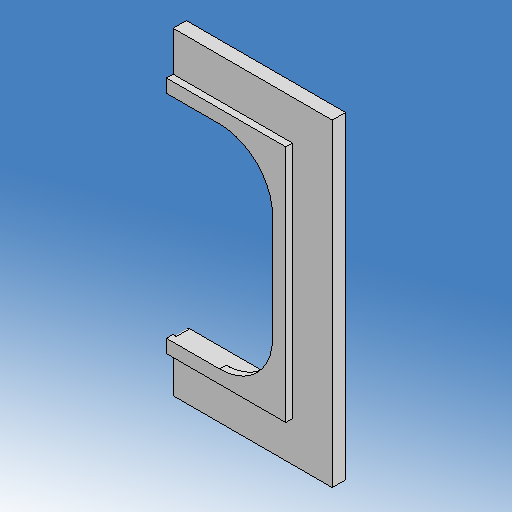
# Autodesk Inventor part: ChassisInterfaceFix
Saved by Autodesk Inventor 2025 (Build 290162000, 162)
## iProperties
Created: 2024-07-07
Part Number: ChassisInterfaceFix
Material: Generic
Document SubType Name: Modeling
Designer: seene
Density: 1 g/cm^3
Appearance: Default
Author: seene
Autodesk Inventor part; units mm, degrees
ref_plane "YZ Plane" through (0, 0, 0) normal (1, 0, 0) x (0, 1, 0)
ref_plane "XZ Plane" through (0, 0, 0) normal (0, 1, 0) x (-1, 0, 0)
ref_plane "XY Plane" through (0, 0, 0) normal (0, 0, 1) x (1, 0, 0)
sketch "Sketch1" plane through (0, 0, 0) normal (0, 0, 1) x (1, 0, 0)
  line L0 (0, 0) -> (76.2, 0)
  line L1 (76.2, 0) -> (76.2, 152.4)
  line L2 (76.2, 152.4) -> (0, 152.4)
  line L3 (0, 152.4) -> (0, 0)
  line L4 (0, 127) -> (50.8, 127)
  line L5 (50.8, 127) -> (50.8, 25.4)
  line L6 (50.8, 25.4) -> (0, 25.4)
  line L7 (0, 25.4) -> (0, 127)
  point P0 (0, 25.4)
  point P1 (76.2, 76.2)
  dimension "d0" = 101.6
  dimension "d1" = 50.8
  dimension "d2" = 25.4
  dimension "d4" = 25.4
  dimension "d9" = 25.4
  constraints: 16 end point, 4 parallel, 2 horizontal, 2 perpendicular, 1 midpoint, 1 point on line
  measures "d0" distance of L4.end L5.end
  measures "d1" distance of L4.start L4.end
  measures "d2" distance between parallel lines of L0 L6
  measures "d4" distance between parallel lines of L4 L2
  measures "d9" distance from line of point (76.2, 76.2) L5
extrude "Extrusion1" add sketch "Sketch1" along normal blind 6.35 contours L3 L6 L5 L4 L2 L1 L0
fillet "Fillet1" radius 12.7 2 edges at (50.8, 127, 3.175) (50.8, 25.4, 3.175)
fillet "Fillet2" radius 1.5875 2 edges at (0, 127, 3.175) (0, 25.4, 3.175)
sketch "Sketch2" plane through (0, 0, 6.35) normal (0, 0, 1) x (1, 0, 0)
  line L0 (0, 127) -> (25.4, 127)
  line L1 (50.8, 101.6) -> (50.8, 50.8)
  line L2 (25.4, 25.4) -> (19.0762, 25.4)
  line L3 (1.5875, 127) -> (38.1, 127) projected
  arc A0 (50.8, 101.6) -> (25.4, 127) centre (25.4, 101.6) ccw
  arc A1 (25.4, 25.4) -> (50.8, 50.8) centre (25.4, 50.8) ccw
  line L4 (38.1, 25.4) -> (1.5875, 25.4) projected
  line L5 (76.2, 0) -> (76.2, 152.4) projected
  line L6 (0, 127) -> (0, 133.35)
  line L7 (0, 133.35) -> (57.15, 133.35)
  line L8 (57.15, 133.35) -> (57.15, 19.05)
  line L9 (57.15, 19.05) -> (0, 19.05)
  line L10 (0, 19.05) -> (0, 25.4)
  line L11 (0, 25.4) -> (1.5875, 25.4)
  line L12 (0, 152.4) -> (0, 128.5875) projected
  line L13 (0, 23.8125) -> (0, 0) projected
  point P0 (0.7937, 25.4)
  dimension "d11" = 25.4
  dimension "d12" = 25.4
  dimension "d13" = 25.4
  dimension "d14" = 6.35
  dimension "d15" = 6.35
  dimension "d16" = 6.35
  constraints: 18 end point, 4 collinear, 4 horizontal, 4 point on circle, 4 tangent, 2 centre point, 2 perpendicular, 2 vertical, 1 midpoint
  measures "d11" radius of A0
  measures "d12" radius of A1
  measures "d13" distance between parallel lines of L5 L1
  measures "d14" distance between parallel lines of L8 L1
  measures "d15" distance between parallel lines of L9 L4
  measures "d16" distance between parallel lines of L0 L7
extrude "Extrusion2" add sketch "Sketch2" along normal blind 3.175
equation "\"d15\" = d14"
equation "\"d16\" = d14"
body "Solid1"
